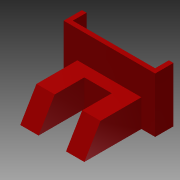
# Autodesk Inventor part: 知能ロボコン発射台支え
Saved by Autodesk Inventor 2013 (Build 170138000, 138)
## iProperties
Created: 2014-05-17
Part Number: 知能ロボコン発射台支え
Material: ABS プラスチック
Document SubType Name: Modeling
Designer: horumo136
Density: 1 g/cm^3
Author: horumo136
Autodesk Inventor part; units mm, degrees
ref_plane "YZ Plane" through (0, 0, 0) normal (1, 0, 0) x (0, 1, 0)
ref_plane "XZ Plane" through (0, 0, 0) normal (0, 1, 0) x (-1, 0, 0)
ref_plane "XY Plane" through (0, 0, 0) normal (0, 0, 1) x (1, 0, 0)
sketch "スケッチ1" plane through (0, 0, 0) normal (1, 0, 0) x (0, 1, 0)
  line L0 (0.6302, 30) -> (-49.0748, 30)
  line L1 (0.6302, 0) -> (-66.7648, 0)
  line L2 (-49.0748, 30) -> (-66.7648, 0)
  line L3 (0.6302, 30) -> (0.6302, 0)
  line L4 (0.6302, 0) -> (0.6302, 30)
  point P0 (0, 0)
  dimension "d0" = 30
  dimension "d30" = 67.395
  dimension "d31" = 49.705
  constraints: 10 end point, 1 perpendicular
  measures "d0" distance between parallel lines of L0 L1
  measures "d30" distance of L1.start L1.end
  measures "d31" distance of L0.start L0.end
extrude "押し出し1" add sketch "スケッチ1" along normal blind 70
sketch "スケッチ7" plane through (0, -66.7648, 0) normal (0, 0, -1) x (-1, 0, 0)
  line L0 (0, 67.395) -> (-70, 67.395) projected
  line L1 (0, 0) -> (-70, 0) projected
  line L2 (-35, 67.395) -> (-35, 0)
  line L3 (-35, 0) -> (-35, 50)
  line L4 (-50, 50) -> (-20, 50)
  line L5 (-20, 50) -> (-20, 0)
  line L6 (-20, 0) -> (-50, 0)
  line L7 (-50, 0) -> (-50, 50)
  line L8 (-50, 50) -> (-20, 0) construction
  line L9 (-20, 50) -> (-50, 0) construction
  point P0 (0, 66.7648)
  point P1 (-35, 25)
  dimension "d32" = 50
  dimension "d33" = 30
  constraints: 16 end point, 5 midpoint, 2 parallel, 2 point on line, 1 horizontal, 1 perpendicular
  measures "d32" distance of L2.end L3.end
  measures "d33" distance of L5.end L6.end
extrude "押し出し4" cut sketch "スケッチ7" against normal blind 50
sketch "スケッチ8" plane through (0, 0.6302, 30) normal (0, 1, 0) x (1, 0, 0)
  line L0 (0, 30) -> (0, 0) projected
  line L1 (0, 0) -> (70, 0) projected
  line L2 (70, 30) -> (70, 0) projected
  line L3 (0, 30) -> (70, 30) projected
  line L4 (-15, 30) -> (85, 30)
  line L5 (85, 30) -> (85, -20)
  line L6 (85, -20) -> (-15, -20)
  line L7 (-15, -20) -> (-15, 30)
  line L8 (-15, 30) -> (85, -20) construction
  line L9 (85, 30) -> (-15, -20) construction
  point P0 (35, 5)
  dimension "d36" = 100
  dimension "d37" = 50
  dimension "d44" = 30
  constraints: 12 end point, 2 midpoint, 2 parallel, 1 horizontal, 1 perpendicular
  measures "d36" distance of L5.end L6.end
  measures "d37" distance of L4.end L5.end
  measures "d44" distance between parallel lines of L1 L4
extrude "押し出し5" add sketch "スケッチ8" against normal blind 5 contours L0 L1 L2 L4 L5 L6 L7
sketch "スケッチ9" plane through (-15, 0.6302, 0) normal (0, 1, 0) x (1, 0, 0)
  line L0 (100, -50) -> (0, -50) projected
  line L1 (0, 0) -> (5, 0)
  line L2 (5, 0) -> (5, -50)
  line L3 (5, -50) -> (0, -50)
  line L4 (0, -50) -> (0, 0)
  line L5 (100, 0) -> (95, 0)
  line L6 (95, 0) -> (95, -50)
  line L7 (95, -50) -> (100, -50)
  line L8 (100, -50) -> (100, 0)
  point P0 (15, 0)
  dimension "d40" = 5
  dimension "d41" = 5
  constraints: 16 end point, 4 parallel, 2 horizontal, 2 perpendicular, 2 point on line
  measures "d40" distance of L2.end L3.end
  measures "d41" distance of L7.end L6.end
extrude "押し出し6" add sketch "スケッチ9" along normal blind 15
sketch "スケッチ10" plane through (-15, -4.3698, 50) normal (0, 0, 1) x (1, 0, 0)
  line L0 (95, 5) -> (5, 5) projected
  line L1 (5, 5) -> (5, 20) projected
  line L2 (0, 20) -> (5, 20) projected
  line L3 (0, 20) -> (0, 0) projected
  line L4 (100, 0) -> (0, 0) projected
  line L5 (100, 20) -> (100, 0) projected
  line L6 (95, 20) -> (100, 20) projected
  line L7 (95, 5) -> (95, 20) projected
  point P0 (15, 4.3698)
extrude "押し出し7" add sketch "スケッチ10" along normal blind 10
